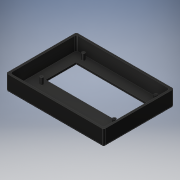
# Autodesk Inventor part: receiver-box
Saved by Autodesk Inventor 2017 (Build 210142000, 142)
## iProperties
Created: 2020-06-15
Part Number: receiver-box
Material: ABS Plastic
Document SubType Name: Modeling
Designer: HAYNIE
Density: 1.06 g/cm^3
Appearance: Glossy - Black
Author: HAYNIE
Autodesk Inventor part; units mm, degrees
ref_plane "YZ Plane" through (0, 0, 0) normal (1, 0, 0) x (0, 1, 0)
ref_plane "XZ Plane" through (0, 0, 0) normal (0, 1, 0) x (-1, 0, 0)
ref_plane "XY Plane" through (0, 0, 0) normal (0, 0, 1) x (1, 0, 0)
sketch "Box-Sketch" plane through (0, 0, 0) normal (0, 1, 0) x (-1, 0, 0)
  line L0 (0.0036, -89.9982) -> (0.0036, 0.0018)
  line L1 (0.0036, 0.0018) -> (-124.9964, 0.0018)
  line L2 (-124.9964, 0.0018) -> (-124.9964, -89.9982)
  line L3 (-124.9964, -89.9982) -> (0.0036, -89.9982)
  point P0 (0, 0)
  dimension "d0" = 90
  dimension "d1" = 125
  constraints: 8 end point, 2 parallel, 1 perpendicular
  measures "d0" distance of L2.end L1.end
  measures "d1" distance of L1.end L0.end
extrude "Box-Extrude" add sketch "Box-Sketch" along normal blind 20
shell "Box-Shell" thickness 2.54 removed faces 1 at (83.3297, 20, -29.9982)
sketch "LCD-Sketch" plane through (2.5364, 2.54, -87.4582) normal (0, 1, 0) x (0, 0, 1)
  line L0 (12.6293, 12.7312) -> (52.1293, 12.7312)
  line L1 (52.1293, 12.7312) -> (52.1293, 109.7312)
  line L2 (52.1293, 109.7312) -> (12.6293, 109.7312)
  line L3 (12.6293, 109.7312) -> (12.6293, 12.7312)
  point P0 (87.4582, -2.5364)
  dimension "d41" = 39.5
  dimension "d42" = 97
  constraints: 8 end point, 2 parallel, 1 horizontal, 1 perpendicular
  measures "d41" distance of L2.end L1.end
  measures "d42" distance of L1.end L0.end
extrude "LCD-Extrude" cut sketch "LCD-Sketch" along normal mid plane 76.2
sketch "LCD-Posts" plane through (2.5364, 2.54, -87.4582) normal (0, 1, 0) x (0, 0, 1)
  circle A0 centre (5.6293, 107.5979) radius 2
  circle A1 centre (59.1293, 107.7876) radius 2
  circle A2 centre (59.1293, 14.7168) radius 2
  circle A3 centre (5.632, 14.7168) radius 2
  constraints: 4 centre point
extrude "Extrusion3" add sketch "LCD-Posts" along normal blind 8
hole "Hole6" at (17.2059, 10.54, -81.7213) direction (0, -1, 0) diameter 1.5 depth 5
hole "Hole7" at (110.1552, 10.54, -81.8394) direction (0, -1, 0) diameter 1.5 depth 5
hole "Hole8" at (110.324, 10.54, -28.3394) direction (0, -1, 0) diameter 1.5 depth 5
hole "Hole9" at (17.2742, 10.54, -28.3395) direction (0, -1, 0) diameter 1.5 depth 5
fillet "Fillet1" radius 2 1 edges at (124.9964, 0, -44.9982)
fillet "Fillet2" radius 2 3 edges at (61.4964, 0, -89.9982) (124.4106, 0.5858, -89.9982) (124.9964, 11, -89.9982)
fillet "Fillet3" radius 2 3 edges at (61.4964, 0, 0.0018) (124.4106, 0.5858, 0.0018) (124.9964, 11, 0.0018)
fillet "Fillet4" radius 2 5 edges at (-0.0036, 0, -44.9982) (-0.0036, 0.5858, -0.584) (-0.0036, 11, 0.0018) (-0.0036, 0.5858, -89.4125) (-0.0036, 11, -89.9982)
fillet "Fillet5" radius 2 1 edges at (2.5364, 11.27, -87.4582)
fillet "Fillet6" radius 2 1 edges at (122.4564, 11.27, -2.5382)
fillet "Fillet7" radius 2 1 edges at (2.5364, 11.27, -2.5382)
fillet "Fillet8" radius 2 1 edges at (122.4564, 11.27, -87.4582)
body "Solid1"
